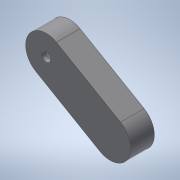
# Autodesk Inventor part: Y belt Cover
Saved by Autodesk Inventor 2020 (Build 240168000, 168)
## iProperties
Created: 2019-06-07
Part Number: Y belt Cover
Material: Generic
Document SubType Name: Modeling
Designer: LillaHunden
Density: 1 g/cm^3
Appearance: Default
Author: LillaHunden
Autodesk Inventor part; units mm, degrees
ref_plane "YZ Plane" through (0, 0, 0) normal (1, 0, 0) x (0, 1, 0)
ref_plane "XZ Plane" through (0, 0, 0) normal (0, 1, 0) x (-1, 0, 0)
ref_plane "XY Plane" through (0, 0, 0) normal (0, 0, 1) x (1, 0, 0)
sketch "Sketch1" plane through (0, 0, 0) normal (0, 0, 1) x (1, 0, 0)
  line L0 (-103.0486, 32.008) -> (-29.0145, -10.8833) construction
  line L1 (-85.2832, 36.7398) -> (-33.7462, 6.8821)
  line L2 (-46.7799, -15.6151) -> (-98.3168, 14.2426)
  arc A0 (-85.2832, 36.7398) -> (-98.3168, 14.2426) centre (-91.8, 25.4912) ccw
  arc A1 (-46.7799, -15.6151) -> (-33.7462, 6.8821) centre (-40.2631, -4.3665) ccw
  circle A2 centre (-91.8, 25.4912) radius 4.5363 construction
  circle A3 centre (-43.5, -2.4912) radius 4.2314 construction
  line L3 (7.6716, 38.4912) -> (-163.6716, 38.4912) construction
  line L4 (-100.0713, 11.2141) -> (-48.5344, -18.6435)
  arc A4 (-48.5344, -18.6435) -> (-31.9917, 9.9106) centre (-40.2631, -4.3665) ccw
  line L5 (-31.9917, 9.9106) -> (-83.5287, 39.7682)
  arc A5 (-83.5287, 39.7682) -> (-100.0713, 11.2141) centre (-91.8, 25.4912) ccw
  point P0 (0, 0)
  point P1 (-66.0315, 10.5623)
  dimension "d0" = 3.5
  constraints: 12 end point, 10 point on circle, 5 tangent, 4 centre point, 4 point on line, 2 parallel, 1 coincident, 1 midpoint, 3 other
  measures "d0" distance between parallel lines of L2 L4
extrude "Extrusion1" add sketch "Sketch1" along normal blind 15.5
sketch "Sketch2" plane through (0, 0, 15.5) normal (0, 0, 1) x (1, 0, 0)
  arc A0 (-83.5287, 39.7682) -> (-100.0713, 11.2141) centre (-91.8, 25.4912) ccw projected
  line L0 (-31.9917, 9.9106) -> (-83.5287, 39.7682) projected
  arc A1 (-48.5344, -18.6435) -> (-31.9917, 9.9106) centre (-40.2631, -4.3665) ccw projected
  line L1 (-100.0713, 11.2141) -> (-48.5344, -18.6435) projected
  point P0 (0, 0)
extrude "Extrusion2" add sketch "Sketch2" along normal blind 3.5
sketch "Sketch3" plane through (0, 0, 19) normal (0, 0, 1) x (1, 0, 0)
  circle A0 centre (-91.8, 25.4912) radius 2.5 construction
  circle A1 centre (-91.8, 25.4912) radius 3.65
  point P0 (0, 0)
  dimension "d5" = 7.3
  constraints: 1 centre point, 1 coincident
  measures "d5" diameter of A1
extrude "Extrusion3" cut sketch "Sketch3" against normal through all
sketch "Sketch4" plane through (0, 0, 0) normal (0, 0, -1) x (-1, 0, 0)
  line L0 (121.4345, 25.6088) -> (42.3921, 25.6088) construction
  arc A0 (115.98, 18.7815) -> (116.2693, 32.3641) centre (114.4345, 25.6088) ccw
  arc A1 (49.3921, 32.6088) -> (49.3921, 18.6088) centre (49.3921, 25.6088) ccw
  circle A2 centre (114.4345, 25.6088) radius 3.5
  circle A3 centre (49.3921, 25.6088) radius 3.5
  line L1 (31.9917, 9.9106) -> (83.5287, 39.7682) projected
  line L2 (100.0713, 11.2141) -> (48.5344, -18.6435) projected
  arc A4 (100.0713, 11.2141) -> (83.5287, 39.7682) centre (91.8, 25.4912) ccw projected
  arc A5 (31.9917, 9.9106) -> (48.5344, -18.6435) centre (40.2631, -4.3665) ccw projected
  line L3 (116.2693, 32.3641) -> (106.8288, 32.3018)
  line L4 (115.98, 18.7815) -> (106.5624, 18.1208)
  line L5 (49.3921, 32.6088) -> (71.1708, 32.6088)
  line L6 (9.0132, -8.6068) -> (88.0556, -8.6068) construction
  line L7 (16.0132, -1.6068) -> (81.0556, -1.6068)
  line L8 (81.0556, -15.6068) -> (16.0132, -15.6068)
  arc A6 (16.0132, -1.6068) -> (16.0132, -15.6068) centre (16.0132, -8.6068) ccw
  arc A7 (81.0556, -15.6068) -> (81.0556, -1.6068) centre (81.0556, -8.6068) ccw
  circle A8 centre (16.0132, -8.6068) radius 3.5
  circle A9 centre (81.0556, -8.6068) radius 3.5
  point P0 (0, 0)
  point P1 (81.9133, 25.6088)
  point P2 (47.47, 18.8779)
  point P3 (48.5344, -8.6068)
  point P4 (77.9414, -1.6068)
  point P5 (53.7761, -15.6068)
  point P6 (28.1839, -15.6068)
  point P7 (23.9955, -1.6068)
  dimension "d8" = 7
  dimension "d9" = 7
  dimension "d12" = 65.0425
  dimension "d13" = 65.0425
  dimension "d14" = 7
  dimension "d15" = 7
  dimension "d16" = 7
  dimension "d17" = 7
  dimension "d18" = 7
  constraints: 18 end point, 14 point on circle, 8 centre point, 6 tangent, 5 point on line, 4 coincident, 2 horizontal, 2 midpoint, 1 equal length, 1 parallel
  measures "d8" diameter of A2
  measures "d9" diameter of A3
  measures "d12" distance of A0.centre A1.centre
  measures "d13" distance of A6.centre A7.centre
  measures "d14" radius of A6
  measures "d15" radius of A1
  measures "d16" radius of A0
  measures "d17" diameter of A8
  measures "d18" diameter of A9
extrude "Extrusion4" add sketch "Sketch4" against normal blind 9.25 contours L4 A4 L3 A0 | L7 A7 L8 L2 | L1 A1 L5 | A5 L8 A6 L7
equation "\"d13\" = d12"
equation "\"d14\" = d15"
equation "\"d16\" = d15"
body "Solid1"
